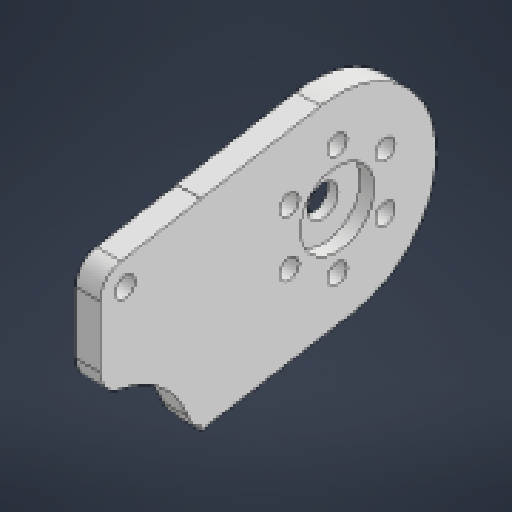
# Autodesk Inventor part: MotorMount
Saved by Autodesk Inventor 2024.2 (Build 282272000, 272)
## iProperties
Created: 2023-12-29
Part Number: MotorMount
Material: 一般
Document SubType Name: Modeling
Designer: Hanaoka
Density: 1 g/cm^3
Appearance: 既定
Author: Hanaoka
Autodesk Inventor part; units mm, degrees
ref_plane "YZ Plane" through (0, 0, 0) normal (1, 0, 0) x (0, 1, 0)
ref_plane "XZ Plane" through (0, 0, 0) normal (0, 1, 0) x (-1, 0, 0)
ref_plane "XY Plane" through (0, 0, 0) normal (0, 0, 1) x (1, 0, 0)
sketch "スケッチ1" plane through (0, 0, 0) normal (1, 0, 0) x (0, 1, 0)
  circle A0 centre (0, 0) radius 3
  circle A1 centre (0, 0) radius 4.5 construction
  circle A2 centre (4.5, 0) radius 0.8
  circle A3 centre (2.25, 3.8971) radius 0.8
  circle A4 centre (-2.25, 3.8971) radius 0.8
  circle A5 centre (-4.5, 0) radius 0.8
  circle A6 centre (-2.25, -3.8971) radius 0.8
  circle A7 centre (2.25, -3.8971) radius 0.8
  line L0 (-25.1126, 0) -> (14.9601, 0) projected
  line L1 (6.2329, 11) -> (-10, 11)
  line L2 (-10, 11) -> (-7.8852, -1.3502)
  circle A8 centre (0, 0) radius 1.25
  line L3 (0, 0) -> (-10, 0) construction
  line L4 (-10, 0) -> (-10, 11) construction
  arc A9 (-7.8852, -1.3502) -> (7.8852, 1.3502) centre (0, 0) ccw
  line L5 (6.2329, 11) -> (7.8852, 1.3502)
  line L6 (-13.5106, 12.8383) -> (-10.0642, 11.2105) projected
  line L7 (-10.0642, 11.2105) -> (-7.9495, -1.1398) projected
  arc A10 (-7.9495, -1.1398) -> (7.821, 1.5607) centre (-0.0642, 0.2105) ccw projected
  line L8 (7.821, 1.5607) -> (5.0943, 17.4845) projected
  arc A11 (5.0943, 17.4845) -> (3.9772, 18.9553) centre (3.123, 17.1469) ccw projected
  line L9 (3.9772, 18.9553) -> (-7.9583, 24.593) projected
  arc A12 (-7.9583, 24.593) -> (-13.5106, 12.8383) centre (-10.7344, 18.7156) ccw projected
  circle A13 centre (-0.0642, 0.2105) radius 1 projected
  circle A14 centre (3.123, 17.1469) radius 0.8 projected
  circle A15 centre (-10.7344, 18.7156) radius 3 projected
  arc A16 (-8.4779, 12.0893) -> (-3.8416, 17.4955) centre (-10.7344, 18.7156) ccw
  line L10 (-1.8722, 19.1469) -> (3.123, 19.1469)
  arc A17 (5.0943, 17.4845) -> (3.123, 19.1469) centre (3.123, 17.1469) ccw
  line L11 (-9.8045, 9.8585) -> (-10, 11)
  arc A18 (-1.8722, 19.1469) -> (-3.8416, 17.4955) centre (-1.8722, 17.1469) ccw
  arc A19 (-8.4779, 12.0893) -> (-9.8045, 9.8585) centre (-7.8332, 10.1961) ccw
  point P0 (7.5963, 0)
  point P1 (-10.1271, 11.742)
  point P2 (-3.7477, 19.1469)
  point P3 (-9.6645, 11)
  point P4 (6.2047, 11)
  point P5 (3.9772, 18.9553)
  dimension "d1" = 9
  dimension "d0" = 6
  dimension "d2" = 1.6
  dimension "d5" = 360
  dimension "d8" = 2.5
  dimension "d13" = 8
  dimension "d14" = 10
  dimension "d15" = 11
  dimension "d16" = 7
  dimension "d17" = 2
  constraints: 14 end point, 13 centre point, 13 point on circle, 7 tangent, 6 point on line, 5 coincident, 3 horizontal, 2 equal radius, 1 collinear, 1 horizontal alignment, 1 parallel, 1 vertical, 15 other
  measures "d0" diameter of A0
  measures "d2" diameter of A2
  measures "d8" diameter of A8
  measures "d13" radius of A9
  measures "d14" distance of L3.start L3.end
  measures "d15" distance of L1.end L3.end
  measures "d16" radius of A16
  measures "d17" radius of A18
extrude "押し出し1" add sketch "スケッチ1" against normal blind 2 contours L0 A8 A0 | L0 A2 A10 A9 L2 A5 A0 | A0 L0 A8 | A0 L0 A5 L2 A19 L1 L8 A10 A2 | A10 L8 L1 L5 A9 L0 | L0 A9 A10 | L2 L1 A19 | L1 A19 A16 A18 L10 A17 A11 L8
extrude "押し出し2" cut sketch "スケッチ1" against normal blind 1.15 contours L0 A8 A0 | A0 L0 A8
